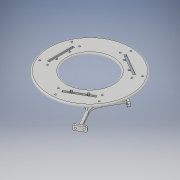
# Autodesk Inventor part: Stewart-Platform-Base-Außenanordnung
Saved by Autodesk Inventor 2018.2 (Build 222227000, 227)
## iProperties
Created: 2018-02-17
Part Number: Stewart-Platform-Base-Außenanordnung
Material: Generisch
Document SubType Name: Modeling
Designer: JochenAlt
Density: 1 g/cm^3
Appearance: Vorgabe
Author: JochenAlt
Autodesk Inventor part; units mm, degrees
ref_plane "YZ Plane" through (0, 0, 0) normal (1, 0, 0) x (0, 1, 0)
ref_plane "XZ Plane" through (0, 0, 0) normal (0, 1, 0) x (-1, 0, 0)
sketch "Skizze1" plane through (0, 0, 0) normal (0, 0, 1) x (1, 0, 0)
  line L0 (0, 93.7804) -> (0, -93.7804) construction
  line L1 (-93.7804, 0) -> (93.7804, 0) construction
  line L2 (-54.7144, 28.85) -> (-42.2144, 28.85) construction
  line L3 (-38.9144, 25.55) -> (-38.9144, -25.55) construction
  line L4 (-42.2144, -28.85) -> (-54.7144, -28.85) construction
  line L5 (-58.0144, -25.55) -> (-58.0144, 25.55) construction
  arc A0 (-54.7144, 28.85) -> (-58.0144, 25.55) centre (-54.7144, 25.55) ccw construction
  arc A1 (-38.9144, 25.55) -> (-42.2144, 28.85) centre (-42.2144, 25.55) ccw construction
  arc A2 (-42.2144, -28.85) -> (-38.9144, -25.55) centre (-42.2144, -25.55) ccw construction
  arc A3 (-58.0144, -25.55) -> (-54.7144, -28.85) centre (-54.7144, -25.55) ccw construction
  circle A4 centre (-54.7144, 25.55) radius 1.3
  circle A5 centre (-42.2144, 25.55) radius 1.3
  circle A6 centre (-54.7144, -25.55) radius 1.3
  circle A7 centre (-42.2144, -25.55) radius 1.3
  line L6 (-44.9144, 20.25) -> (-44.9144, -20.25)
  line L7 (-48.0144, 20.25) -> (-48.0144, -20.25)
  line L8 (-48.0144, 20.25) -> (-44.9144, 20.25)
  line L9 (-48.0144, -20.25) -> (-44.9144, -20.25)
  line L10 (-48.0144, 0.8) -> (-44.9144, 0.8)
  line L11 (-48.0144, -0.8) -> (-44.9144, -0.8)
  line L12 (-44.9144, 11.55) -> (-41.8984, 11.55)
  line L13 (-41.8984, 11.55) -> (-41.8984, 8.75)
  line L14 (-41.8984, 8.75) -> (-44.9144, 8.75)
  line L15 (-44.9144, -8.75) -> (-41.8984, -8.75)
  line L16 (-41.8984, -8.75) -> (-41.8984, -11.55)
  line L17 (-41.8984, -11.55) -> (-44.9144, -11.55)
  line L18 (-42.2144, 29.15) -> (-54.7144, 29.15)
  arc A8 (-54.7144, 29.15) -> (-58.3144, 25.55) centre (-54.7144, 25.55) ccw
  line L19 (-58.3144, 25.55) -> (-58.3144, -25.55)
  arc A9 (-58.3144, -25.55) -> (-54.7144, -29.15) centre (-54.7144, -25.55) ccw
  line L20 (-54.7144, -29.15) -> (-42.2144, -29.15)
  arc A10 (-42.2144, -29.15) -> (-38.6144, -25.55) centre (-42.2144, -25.55) ccw
  line L21 (-38.6144, -25.55) -> (-38.6144, 25.55)
  arc A11 (-38.6144, 25.55) -> (-42.2144, 29.15) centre (-42.2144, 25.55) ccw
  line L22 (-60.4453, -28.8235) -> (-57.8404, -27.3356) construction
  line L23 (-35.6144, 0) -> (-38.6144, 0) construction
  circle A12 centre (0, 0) radius 35.6144
  circle A13 centre (0, 0) radius 66.986
  line L24 (-60.6945, 28.3425) -> (-57.9762, 27.0732) construction
  line L25 (-41.8984, -10.15) -> (-5.8601, -10.15) construction
  line L26 (6.3855, -31.3601) -> (-5.8601, -10.15) construction
  line L27 (-37.6144, -10.15) -> (-37.6144, -65.15) construction
  line L28 (10.017, -37.65) -> (-37.6144, -65.15) construction
  line L29 (-38.6144, -19.95) -> (-44.9144, -19.95)
  line L30 (-38.6144, 19.95) -> (-44.9144, 19.95)
  arc A14 (46.3518, -21.9837) -> (41.4341, -20.666) centre (43.2341, -23.7837) ccw
  circle A15 centre (43.2341, -23.7837) radius 1.3
  line L31 (41.4341, -20.666) -> (-2.8198, -46.216)
  line L32 (36.5844, -23.466) -> (39.7344, -28.922)
  line L33 (30.9518, -30.5101) -> (32.4598, -33.122)
  line L34 (28.5269, -31.9101) -> (30.9518, -30.5101)
  line L35 (30.0349, -34.522) -> (28.5269, -31.9101)
  line L36 (4.9202, -49.022) -> (39.9942, -28.772)
  line L37 (41.5442, -31.4567) -> (39.9942, -28.772)
  line L38 (6.4702, -51.7067) -> (41.5442, -31.4567)
  line L39 (24.7, -41.1817) -> (23.15, -38.497)
  line L40 (23.3144, -41.9817) -> (21.7644, -39.297)
  line L41 (10.9466, -42.0601) -> (13.3715, -40.6601)
  line L42 (13.3715, -40.6601) -> (14.8795, -43.272)
  line L43 (12.4546, -44.672) -> (10.9466, -42.0601)
  line L44 (2.03, -43.416) -> (5.18, -48.872)
  line L45 (6.4702, -51.7067) -> (4.9202, -49.022)
  arc A16 (-2.8198, -46.216) -> (-4.1375, -51.1337) centre (-1.0198, -49.3337) ccw
  circle A17 centre (-1.0198, -49.3337) radius 1.3
  line L46 (-4.1375, -51.1337) -> (2.1125, -61.959)
  circle A18 centre (49.4841, -34.609) radius 1.3
  arc A19 (51.2841, -37.7267) -> (52.6018, -32.809) centre (49.4841, -34.609) ccw
  line L47 (7.0302, -63.2767) -> (51.2841, -37.7267)
  circle A20 centre (5.2302, -60.159) radius 1.3
  arc A21 (2.1125, -61.959) -> (7.0302, -63.2767) centre (5.2302, -60.159) ccw
  line L48 (52.6018, -32.809) -> (46.3518, -21.9837)
  arc A22 (-4.1375, 51.1337) -> (-2.8198, 46.216) centre (-1.0198, 49.3337) ccw
  circle A23 centre (-1.0198, 49.3337) radius 1.3
  line L49 (-2.8198, 46.216) -> (41.4341, 20.666)
  line L50 (2.03, 43.416) -> (5.18, 48.872)
  line L51 (10.9466, 42.0601) -> (12.4546, 44.672)
  line L52 (13.3715, 40.6601) -> (10.9466, 42.0601)
  line L53 (14.8795, 43.272) -> (13.3715, 40.6601)
  line L54 (39.9942, 28.772) -> (4.9202, 49.022)
  line L55 (6.4702, 51.7067) -> (4.9202, 49.022)
  line L56 (41.5442, 31.4567) -> (6.4702, 51.7067)
  line L57 (23.3144, 41.9817) -> (21.7644, 39.297)
  line L58 (24.7, 41.1817) -> (23.15, 38.497)
  line L59 (30.9518, 30.5101) -> (28.5269, 31.9101)
  line L60 (28.5269, 31.9101) -> (30.0349, 34.522)
  line L61 (32.4598, 33.122) -> (30.9518, 30.5101)
  line L62 (36.5844, 23.466) -> (39.7344, 28.922)
  line L63 (41.5442, 31.4567) -> (39.9942, 28.772)
  arc A24 (41.4341, 20.666) -> (46.3518, 21.9837) centre (43.2341, 23.7837) ccw
  circle A25 centre (43.2341, 23.7837) radius 1.3
  line L64 (46.3518, 21.9837) -> (52.6018, 32.809)
  circle A26 centre (5.2302, 60.159) radius 1.3
  arc A27 (7.0302, 63.2767) -> (2.1125, 61.959) centre (5.2302, 60.159) ccw
  line L65 (51.2841, 37.7267) -> (7.0302, 63.2767)
  circle A28 centre (49.4841, 34.609) radius 1.3
  arc A29 (52.6018, 32.809) -> (51.2841, 37.7267) centre (49.4841, 34.609) ccw
  line L66 (2.1125, 61.959) -> (-4.1375, 51.1337)
  point P0 (0, 2)
  point P1 (0, -2)
  point P2 (-38.6144, -21.4)
  point P3 (-38.6144, 21.4)
  point P4 (19.3072, -33.441)
  point P5 (37.8401, -22.741)
  point P6 (0.7742, -44.141)
  point P7 (29.7393, -31.2101)
  point P8 (52.5935, -36.4234)
  point P9 (5.542, -63.7455)
  point P10 (19.3072, 33.441)
  point P11 (0.7742, 44.141)
  point P12 (37.8401, 22.741)
  point P13 (12.159, 41.3601)
  point P14 (5.2469, 63.759)
  point P15 (52.4342, 36.6723)
  dimension "d43" = 133.9719
  dimension "d1" = 57.7
  dimension "d2" = 19.1
  dimension "d3" = 3.3
  dimension "d5" = 2.6
  dimension "d6" = 6
  dimension "d7" = 3.1
  dimension "d9" = 1.6
  dimension "d10" = 2.984
  dimension "d11" = 2.8
  dimension "d12" = 17.5
  dimension "d21" = 0.3
  dimension "d22" = 3
  dimension "d34" = 3
  dimension "d35" = 3
  dimension "d40" = 1
  dimension "d42" = 55
  dimension "d105" = 360
  dimension "d107" = 40.5
  dimension "d108" = 0.3
  dimension "d109" = 1
  constraints: 124 end point, 38 point on circle, 28 centre point, 23 point on line, 13 coincident, 11 horizontal, 8 tangent, 6 equal radius, 6 perpendicular, 4 midpoint, 4 parallel, 2 line through centre, 2 vertical, 1 collinear, 1 horizontal alignment, 257 other
  measures "d1" distance between parallel lines of L4 L2
  measures "d2" distance between parallel lines of L3 L5
  measures "d3" radius of A0
  measures "d5" diameter of A4
  measures "d9" distance between parallel lines of L11 L10
  measures "d10" distance between parallel lines of L3 L13
  measures "d11" distance between parallel lines of L14 L12
  measures "d12" distance between parallel lines of L15 L14
  measures "d21" distance between parallel lines of L19 L5
  measures "d22" distance of L22.end L22.start
  measures "d34" distance of L23.start L23.end
  measures "d35" distance of L24.start L24.end
  measures "d40" distance between parallel lines of L21 L27
  measures "d42" distance from line of L25 L27.end
  measures "d107" distance between parallel lines of L8 L9
  measures "d108" distance between parallel lines of L29 L9
  measures "d109" distance between parallel lines of L28 L31
extrude "Extrusion5" add sketch "Skizze1" along normal blind 4 contours L8 L7 L9 L6 L29 L21 A10 L20 A9 L19 A8 L18 A11 L30 | L30 L21 L29 L6 L17 L16 L15 L14 L13 L12 | A13 | L48 A19 L47 A21 L46 A16 L31 L44 L36 L45 L38 L37 L32 A14 | L32 L36 L33 L34 L35 L42 L41 L43 L44 L31 | L66 A27 L65 A29 L64 A24 L49 L62 L54 L63 L56 L55 L50 A22 | L50 L54 L51 L52 L53 L60 L59 L61 L62 L49
extrude "Extrusion4" cut sketch "Skizze1" along normal blind 2 contours L8 L7 L9 L6 L29 L21 A10 L20 A9 L19 A8 L18 A11 L30 | L48 A19 L47 A21 L46 A16 L31 L44 L36 L45 L38 L37 L32 A14 | L66 A27 L65 A29 L64 A24 L49 L62 L54 L63 L56 L55 L50 A22
ref_plane "Arbeitsebene2" through (0, 0, -41.8) normal (0, 0, 1) x (1, 0, 0)
sketch "Skizze6" plane through (0, 0, -41.8) normal (0, 0, 1) x (1, 0, 0)
  line L0 (-44.9144, 8.75) -> (-44.9144, -8.75) construction
  line L1 (-44.9144, -8.75) -> (-41.8984, -8.75) construction
  line L2 (-41.8984, -8.75) -> (-41.8984, -11.55) construction
  line L3 (-41.8984, -11.55) -> (-44.9144, -11.55) construction
  line L4 (-44.9144, -11.55) -> (-44.9144, -20.25) construction
  line L5 (-44.9144, -20.25) -> (-48.0144, -20.25) construction
  line L6 (-48.0144, -20.25) -> (-48.0144, 20.25) construction
  line L7 (-44.9144, 20.25) -> (-44.9144, 11.55) construction
  line L8 (-44.9144, 11.55) -> (-41.8984, 11.55) construction
  line L9 (-41.8984, 11.55) -> (-41.8984, 8.75) construction
  line L10 (-41.8984, 8.75) -> (-44.9144, 8.75) construction
  line L11 (-48.0144, 20.25) -> (-44.9144, 20.25) construction
  circle A0 centre (-42.2144, -25.55) radius 1.3 construction
  circle A1 centre (-54.7144, -25.55) radius 1.3 construction
  circle A2 centre (-42.2144, 25.55) radius 1.3 construction
  circle A3 centre (-54.7144, 25.55) radius 1.3 construction
  circle A4 centre (0, 0) radius 35.6144 construction
  circle A5 centre (0, 0) radius 66.986 construction
  line L12 (-44.9144, -8.75) -> (-44.9144, 8.75)
  line L13 (-44.9144, -8.75) -> (-41.8984, -8.75)
  line L14 (-44.9144, 8.75) -> (-44.9144, -8.75) projected
  line L15 (-97.4588, 0) -> (97.4588, 0) construction
  line L16 (0, 97.4588) -> (0, -97.4588) construction
  line L17 (-41.8984, 8.75) -> (-41.8984, 2)
  line L18 (-41.8984, -2) -> (-41.8984, -8.75)
  line L19 (0, 0) -> (-8.9019, -15.4186) construction
  line L20 (0, 0) -> (-9.1171, 15.7912) construction
  arc A6 (-2.7017, -4.6795) -> (-12.7017, -2) centre (-12.7017, -22) ccw
  arc A7 (-12.7017, 2) -> (-2.7017, 4.6795) centre (-12.7017, 22) ccw
  line L21 (-2.7017, -4.6795) -> (0, -6.2393)
  line L22 (-2.7017, 4.6795) -> (0, 6.2393)
  line L23 (-41.8984, -2) -> (-12.7017, -2)
  line L24 (-41.8984, 2) -> (-12.7017, 2)
  line L25 (-41.8984, 8.75) -> (-44.9144, 8.75) projected
  line L26 (-44.9144, 8.75) -> (-41.8984, 8.75)
  arc A8 (0, 1.65) -> (0, -1.65) centre (0, 0) ccw
  line L27 (0, -6.2393) -> (0, -1.65)
  line L28 (0, 1.65) -> (0, 6.2393)
  point P0 (-33.3674, -0.8)
  dimension "d73" = 120
  dimension "d89" = 20
  dimension "d90" = 4
  dimension "d91" = 3.3
  constraints: 26 end point, 6 point on circle, 6 point on line, 5 perpendicular, 4 tangent, 3 centre point, 2 parallel, 1 coincident, 1 collinear, 1 symmetric about line, 1 vertical, 3 other
  measures "d73" angle of L20 L19
  measures "d89" radius of A7
  measures "d90" distance between parallel lines of L23 L24
  measures "d91" diameter of A8
extrude "Extrusion9" add sketch "Skizze6" against normal blind 7.1 separate body
sketch "Skizze7" plane through (-44.9144, -8.75, -41.8) normal (-1, 0, 0) x (0, 0, -1)
  circle A0 centre (3.8, -3.7) radius 1.3
  circle A1 centre (3.8, -13.8) radius 1.3
  line L0 (0, -17.5) -> (0, 0) construction
  line L1 (0, -8.75) -> (7.1, -8.75) construction
  line L2 (7.1, 0) -> (7.1, -17.5) construction
  point P0 (-41.8, -8.75)
  dimension "d76" = 2.6
  dimension "d77" = 10.1
  dimension "d88" = 3.3
  constraints: 2 centre point, 2 end point, 2 midpoint, 1 equal radius, 1 symmetric about line
  measures "d76" diameter of A1
  measures "d77" distance of A0.centre A1.centre
  measures "d88" distance from line of A0.centre L2
extrude "Extrusion10" cut sketch "Skizze7" against normal blind 10 bodies 1 2
pattern_circular "Runde Anordnung5" count 3 over 360 about axis through (0, 0, -10) along (0, 0, 1) of "Extrusion10", "Extrusion9" bodies 2
fillet "Rundung1" radius 2 30 edges at (-2.7017, -4.6795, -41.8) (-27.3, -2, -41.8) (11.918, -24.6425, -41.8) (-2.7017, 4.6795, -41.8) (11.918, 24.6425, -41.8) (-27.3, 2, -41.8) (15.3821, 22.6425, -41.8) (15.3821, -22.6425, -41.8) (5.4034, 0, -41.8) (-2.7017, -4.6795, -48.9) (-27.3, -2, -48.9) (11.918, -24.6425, -48.9) (15.3821, -22.6425, -48.9) (15.3821, 22.6425, -48.9) (5.4034, 0, -48.9) (-43.4064, 8.75, -48.9) (-43.4064, -8.75, -48.9) (14.1255, 41.966, -48.9) (29.2809, 33.216, -48.9) (29.2809, 33.216, -41.8) (14.1255, 41.966, -41.8) (-43.4064, 8.75, -41.8) (-43.4064, -8.75, -41.8) (14.1255, -41.966, -41.8) (14.1255, -41.966, -48.9) (29.2809, -33.216, -41.8) (29.2809, -33.216, -48.9) (11.918, 24.6425, -48.9) (-27.3, 2, -48.9) (-2.7017, 4.6795, -48.9)
fillet "Rundung2" radius 2 4 edges at (-66.986, 0, 4) (-66.986, 0, 0) (-35.6144, 0, 0) (-35.6144, 0, 4)
equation "\"d22\" = d20"
equation "\"d35\" = d34"
equation "\"d44\" = d21"
equation "\"d20\" = 3"
